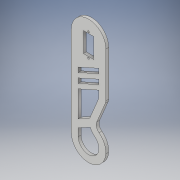
# Autodesk Inventor part: Pata - Brazo
Saved by Autodesk Inventor 2019 (Build 230136000, 136)
## iProperties
Created: 2020-02-12
Part Number: Pata - Brazo
Material: Generic
Document SubType Name: Modeling
Designer: jacqu
Density: 1 g/cm^3
Appearance: Default
Author: jacqu
Autodesk Inventor part; units mm, degrees
ref_plane "YZ Plane" through (0, 0, 0) normal (1, 0, 0) x (0, 1, 0)
ref_plane "XZ Plane" through (0, 0, 0) normal (0, 1, 0) x (-1, 0, 0)
ref_plane "XY Plane" through (0, 0, 0) normal (0, 0, 1) x (1, 0, 0)
sketch "Sketch1" plane through (0, 0, 0) normal (0, 0, 1) x (1, 0, 0)
  arc A0 (20, 0) -> (-20, 0) centre (0, 0) ccw
  line L0 (-20, 0) -> (-20, -104)
  line L1 (20, 0) -> (20, -52)
  arc A1 (19.4895, -54.5451) -> (20, -52) centre (13.4, -52) ccw
  arc A2 (-20, -104) -> (-7.0525, -122.7153) centre (0, -104) ccw
  arc A3 (-7.0525, -122.7153) -> (19.963, -105.2168) centre (0, -104) ccw
  arc A4 (19.963, -105.2168) -> (12.0286, -88.0215) centre (0, -104) ccw
  arc A5 (9.4588, -78.5451) -> (12.0286, -88.0215) centre (16.84, -81.6301) ccw
  line L2 (9.4588, -78.5451) -> (19.4895, -54.5451)
  line L3 (-6, 5.5) -> (6, 5.5)
  line L4 (6, 5.5) -> (6, -17.5)
  line L5 (6, -17.5) -> (-6, -17.5)
  line L6 (-6, -17.5) -> (-6, 5.5)
  circle A6 centre (0, -104) radius 12.5
  dimension "d3" = 20
  dimension "d5" = 52
  dimension "d6" = 20
  dimension "d7" = 20
  dimension "d8" = 8
  dimension "d10" = 6.6
  dimension "d11" = 24
  dimension "d17" = 12
  dimension "d18" = 23
  dimension "d19" = 6
  dimension "d20" = 104
  dimension "d30" = 5.5
  dimension "d39" = 25
  constraints: 14 end point, 13 point on circle, 8 tangent, 7 centre point, 3 parallel, 2 coincident, 1 concentric, 1 horizontal, 1 perpendicular, 1 vertical alignment
  measures "d3" radius of A0
  measures "d5" distance of L1.start L1.end
  measures "d6" radius of A2
  measures "d7" radius of A4
  measures "d8" radius of A5
  measures "d10" radius of A1
  measures "d11" vertical distance of L2.start L2.end
  measures "d17" distance of L3.start L3.end
  measures "d18" distance of L3.end L4.end
  measures "d19" distance from line of L6 point (0, 0)
  measures "d20" distance of L0.start L0.end
  measures "d30" distance from line of point (0, 0) L3
  measures "d39" diameter of A6
extrude "Extrusion1" add sketch "Sketch1" along normal blind 3.3 contours L1 A1 L2 A5 A4 A3 A2 L0 A0 | A6
sketch "Sketch2" plane through (0, 0, 3.3) normal (0, 0, 1) x (1, 0, 0)
  line L0 (-6, 5.5) -> (6, 5.5) projected
  line L1 (6, -17.5) -> (-6, -17.5) projected
  circle A0 centre (0, 7.25) radius 1
  circle A1 centre (0, -19.25) radius 1
  point P0 (0, 0)
  dimension "d31" = 2
  dimension "d32" = 2
  dimension "d34" = 1.75
  dimension "d36" = 1.75
  constraints: 2 centre point, 2 vertical alignment
  measures "d31" diameter of A0
  measures "d32" diameter of A1
  measures "d34" distance from line of L0 A0.centre
  measures "d36" distance from line of L1 A1.centre
extrude "Extrusion2" cut sketch "Sketch2" against normal blind 3.3
sketch "Sketch3" plane through (0, 0, 3.3) normal (0, 0, 1) x (1, 0, 0)
  line L0 (-20, 0) -> (-20, -104) projected
  circle A0 centre (0, 7.25) radius 1 projected
  circle A1 centre (0, -19.25) radius 1 projected
  line L1 (6, 5.5) -> (6, -17.5) projected
  line L2 (6, -17.5) -> (-6, -17.5) projected
  line L3 (-6, -17.5) -> (-6, 5.5) projected
  line L4 (-6, 5.5) -> (6, 5.5) projected
  line L5 (-20, 0) -> (-20, -104) projected
  arc A2 (-20, -104) -> (19.963, -105.2168) centre (0, -104) ccw projected
  arc A3 (9.4588, -78.5451) -> (12.0286, -88.0215) centre (16.84, -81.6301) ccw projected
  line L6 (9.4588, -78.5451) -> (19.4895, -54.5451) projected
  arc A4 (19.4895, -54.5451) -> (20, -52) centre (13.4, -52) ccw projected
  line L7 (20, -52) -> (20, 0) projected
  arc A5 (20, 0) -> (-20, 0) centre (0, 0) ccw projected
  line L8 (-12, -86) -> (-12, -56)
  line L9 (12, -45.2979) -> (12, -53.2979)
  line L10 (12, -53.2979) -> (1.448, -78.5451)
  line L11 (1.448, -78.5451) -> (-12, -86)
  line L12 (9.4588, -78.5451) -> (19.4895, -54.5451) projected
  line L13 (-12, -95.147) -> (-12, -104)
  arc A6 (-12, -104) -> (7.2172, -94.4129) centre (0, -104) ccw
  arc A7 (-20, -104) -> (12.0286, -88.0215) centre (0, -104) ccw projected
  arc A8 (1.9269, -87.4266) -> (7.2172, -94.4129) centre (16.84, -81.6301) ccw
  arc A9 (9.4588, -78.5451) -> (12.0286, -88.0215) centre (16.84, -81.6301) ccw projected
  line L14 (1.9269, -87.4266) -> (-12, -95.147)
  line L15 (-12, -56) -> (12, -45.2979)
  line L16 (-12, -50.5254) -> (12, -39.8233)
  line L17 (12, -39.8233) -> (12, -34.3487)
  line L18 (12, -34.3487) -> (-12, -45.0508)
  line L19 (-12, -45.0508) -> (-12, -50.5254)
  line L20 (-12, -39.5762) -> (12, -28.8741)
  line L21 (12, -28.8741) -> (12, -23.3995)
  line L22 (12, -23.3995) -> (-12, -34.1016)
  line L23 (-12, -39.5762) -> (-12, -34.1016)
  arc A10 (19.963, -105.2168) -> (12.0286, -88.0215) centre (0, -104) ccw projected
  point P0 (19.8711, -53.2979)
  dimension "d45" = 8
  dimension "d46" = 8
  dimension "d48" = 8
  dimension "d49" = 18
  dimension "d52" = 5
  dimension "d53" = 5
  dimension "d54" = 5
  dimension "d55" = 5
  dimension "d56" = 30
  dimension "d57" = 8
  constraints: 30 end point, 8 parallel, 5 point on circle, 4 point on line, 4 vertical, 3 vertical alignment, 2 centre point, 2 concentric, 2 horizontal alignment, 2 tangent
  measures "d45" distance between parallel lines of L8 L0
  measures "d46" distance between parallel lines of L7 L9
  measures "d48" distance from line of L8.start L14
  measures "d49" vertical distance of L0.end L8.start
  measures "d52" distance between parallel lines of L15 L16
  measures "d53" distance between parallel lines of L18 L20
  measures "d54" distance between parallel lines of L16 L18
  measures "d55" distance between parallel lines of L20 L22
  measures "d56" distance of L8.start L8.end
  measures "d57" distance of L9.start L9.end
extrude "Extrusion4" cut sketch "Sketch3" against normal blind 10 contours L8 L15 L9 L10 L11 | L14 A8 A6 L13 | L19 L18 L17 L16 | L23 L22 L21 L20
equation "\"d3\" = radio_muslo"
equation "\"d6\" = radio_muslo"
equation "\"d7\" = d6"
equation "\"d17\" = base_servo"
equation "\"d18\" = altura_servo"
equation "\"d19\" = 0.5 * base_servo"
equation "\"d20\" = 2 * d5"
equation "\"d22\" = espesor"
equation "\"d31\" = agujero_servo"
equation "\"d32\" = agujero_servo"
equation "\"d34\" = distancia_agujero_servo"
equation "\"d36\" = distancia_agujero_servo"
equation "\"d37\" = espesor"
equation "\"espesor\" = 3.3"
equation "\"radio_muslo\" = 20"
equation "\"base_servo\" = 12"
equation "\"altura_servo\" = 23"
equation "\"agujero_servo\" = 2"
equation "\"distancia_agujero_servo\" = 1.75"
body "Solid1"
